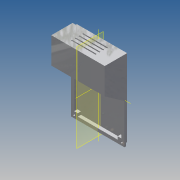
# Autodesk Inventor part: deksel
Saved by Autodesk Inventor 2020.4 (Build 244396000, 396)
## iProperties
Created: 2022-05-18
Part Number: deksel
Material: PC/ABS Plastic
Document SubType Name: Modeling
Designer: Lukas
Density: 0.357273 g/cm^3
Appearance: Smooth - White
Author: Lukas
Autodesk Inventor part; units mm, degrees
ref_plane "XZ Plane" through (0, 0, 0) normal (0, 1, 0) x (-1, 0, 0)
ref_plane "XY Plane" through (0, 0, 0) normal (0, 0, 1) x (1, 0, 0)
sketch "Sketch1" plane through (0, 0, 0) normal (0, 0, 1) x (1, 0, 0)
  line L0 (0, 105) -> (0, -105) projected
  line L1 (-70, 0) -> (70, 0) projected
  line L2 (-50, 75) -> (50, 75)
  line L3 (50, 75) -> (50, -75)
  line L4 (50, -75) -> (-50, -75)
  line L5 (-50, -75) -> (-50, 75)
  line L6 (-44, 69) -> (44, 69)
  line L7 (44, 69) -> (44, -69)
  line L8 (44, -69) -> (-44, -69)
  line L9 (-44, -69) -> (-44, 69)
  point P0 (0, 75)
  point P1 (50, 0)
  dimension "d1" = 100
  dimension "d2" = 150
  dimension "d3" = 6
  dimension "d4" = 6
  dimension "d5" = 6
  dimension "d6" = 6
  constraints: 16 end point, 4 parallel, 2 horizontal, 2 midpoint, 2 perpendicular, 2 point on line
  measures "d1" distance of L3.end L4.end
  measures "d2" distance of L2.end L3.end
  measures "d3" distance between parallel lines of L2 L6
  measures "d4" distance between parallel lines of L3 L7
  measures "d5" distance between parallel lines of L5 L9
  measures "d6" distance between parallel lines of L4 L8
extrude "Extrusion1" add sketch "Sketch1" along normal mid plane 3 contours L2 L3 L1 L7 L6 L0 | L0 L6 L9 L1 L5 L2 | L1 L9 L8 L0 L4 L5 | L3 L4 L0 L8 L7 L1
sketch "Sketch2" plane through (0, 0, -1.5) normal (0, 0, -1) x (-1, 0, 0)
  line L0 (-44, -69) -> (-44, 69) construction
  line L1 (-44, 69) -> (44, 69) construction
  line L2 (44, 69) -> (44, -69) construction
  line L3 (44, -69) -> (-44, -69) construction
  line L4 (44, -69) -> (44, 69) construction
  line L5 (-44, 69) -> (44, 69)
  line L6 (44, 69) -> (44, -69)
  line L7 (44, -69) -> (-44, -69)
  line L8 (-44, -69) -> (-44, 69)
  line L9 (47, -72) -> (-47, -72)
  line L10 (-47, -72) -> (-47, 72)
  line L11 (-47, 72) -> (47, 72)
  line L12 (47, 72) -> (47, -72)
  point P0 (0, 0)
  dimension "d9" = 3
  dimension "d10" = 3
  dimension "d11" = 3
  dimension "d12" = 3
  constraints: 16 end point, 4 parallel, 2 horizontal, 2 perpendicular
  measures "d9" distance between parallel lines of L11 L1
  measures "d10" distance between parallel lines of L10 L0
  measures "d11" distance between parallel lines of L12 L2
  measures "d12" distance between parallel lines of L3 L9
extrude "Extrusion2" add sketch "Sketch2" along normal blind 5
sketch "Sketch4" plane through (50, -75, 1.5) normal (1, 0, 0) x (0, 0, -1)
  line L0 (0, 0) -> (0, 150) construction
  line L1 (0, 0) -> (45, 0) construction
  line L2 (0, 150) -> (0, 0) construction
  line L3 (0, 75) -> (-36.8618, 100.8109)
  line L4 (0, 75) -> (45, 75) construction
  line L5 (0, 150) -> (-36.8618, 150)
  line L6 (-36.8618, 150) -> (-36.8618, 100.8109)
  line L7 (0, 75) -> (0, 150)
  line L8 (3, 0) -> (3, 150) construction
  line L9 (-3, 147) -> (-33.8618, 147)
  line L10 (-33.8618, 147) -> (-33.8618, 102.3726)
  line L11 (-33.8618, 102.3726) -> (-3, 80.7629)
  line L12 (-3, 147) -> (-3, 80.7629)
  line L13 (3, 0) -> (0, 0) construction
  line L14 (0, 78.6623) -> (3, 78.6623)
  line L15 (3, 78.6623) -> (3, 0)
  line L16 (3, 0) -> (0, 0)
  line L17 (0, 0) -> (0, 78.6623)
  point P0 (1.5, 75)
  dimension "d27" = 45
  dimension "d28" = 145
  dimension "d29" = 3
  dimension "d30" = 3
  dimension "d31" = 3
  dimension "d32" = 3
  constraints: 28 end point, 4 horizontal, 4 parallel, 4 perpendicular, 1 equal length, 1 midpoint, 1 point on line, 1 vertical
  measures "d27" distance of L3.start L3.end
  measures "d28" angle of L4 L3
  measures "d29" distance between parallel lines of L6 L10
  measures "d30" distance between parallel lines of L5 L9
  measures "d31" distance between parallel lines of L12 L0
  measures "d32" distance between parallel lines of L3 L11
extrude "Extrusion4" add sketch "Sketch4" against normal blind 100 contours L3 L6 L5 L7
sketch "Sketch5" plane through (47, -72, -1.5) normal (1, 0, 0) x (0, 0, -1)
  line L0 (0, 144) -> (0, 0) construction
  line L1 (5, 0) -> (5, 144) construction
  line L2 (0, 77.7875) -> (5, 77.7875)
  line L3 (5, 77.7875) -> (5, 0)
  line L4 (5, 0) -> (0, 0)
  line L5 (0, 0) -> (0, 77.7875)
  point P0 (-1.5, 72)
  constraints: 8 end point, 2 parallel, 1 horizontal, 1 perpendicular, 1 point on line
extrude "Extrusion5" add sketch "Sketch5" against normal blind 94
sketch "Sketch6" plane through (-44, 5.7875, -1.5) normal (0, 0, 1) x (1, 0, 0)
  line L0 (88, -74.7875) -> (0, -74.7875) construction
  line L1 (88, -5.7875) -> (0, -5.7875) construction
  line L2 (0, -74.7875) -> (88, -74.7875)
  line L3 (88, -74.7875) -> (88, -5.7875)
  line L4 (88, -5.7875) -> (0, -5.7875)
  line L5 (0, -5.7875) -> (0, -74.7875)
  point P0 (44, -5.7875)
  constraints: 8 end point, 2 parallel, 1 horizontal, 1 perpendicular
extrude "Extrusion6" cut sketch "Sketch6" against normal blind 3
sketch "Sketch7" plane through (50, -75, -1.5) normal (1, 0, 0) x (0, 0, -1)
  line L0 (-39.8618, 100.8109) -> (-3, 75) construction
  line L1 (-39.8618, 100.8109) -> (-39.8618, 150) construction
  line L2 (-3, 144) -> (-3, 75) construction
  line L3 (-39.8618, 150) -> (-3, 150)
  line L4 (-3, 150) -> (-3, 100.8109)
  line L5 (-39.8618, 100.8109) -> (-39.8618, 150)
  line L6 (-3, 75) -> (-39.8618, 100.8109) construction
  line L7 (-39.8618, 100.8109) -> (-3, 75)
  line L8 (-3, 75) -> (-3, 100.8109)
  point P0 (-1.5, 75)
  constraints: 10 end point, 2 equal length, 1 horizontal, 1 perpendicular, 1 point on line
extrude "Extrusion7" add sketch "Sketch7" against normal blind 1
sketch "Sketch8" plane through (44, 0, 1.5) normal (0, 0, -1) x (-1, 0, 0)
  line L0 (0, 5.7875) -> (0, 69) construction
  line L1 (88, 69) -> (0, 69)
  line L2 (0, 69) -> (0, 5.7875)
  line L3 (0, 5.7875) -> (88, 5.7875)
  line L4 (88, 5.7875) -> (88, 69)
  point P0 (44, 0)
  constraints: 8 end point, 2 parallel, 1 horizontal, 1 perpendicular
extrude "Extrusion8" cut sketch "Sketch8" against normal blind 3
sketch "Sketch9" plane through (-44, 5.7875, -1.5) normal (0, 0, 1) x (1, 0, 0)
  line L0 (88, -5.7875) -> (0, -5.7875) construction
  line L1 (88, -5.7875) -> (0, -5.7875)
  line L2 (0, -5.7875) -> (0, 0)
  line L3 (0, 0) -> (88, 0)
  line L4 (88, 0) -> (88, -5.7875)
  point P0 (44, -5.7875)
  constraints: 8 end point, 2 parallel, 1 horizontal, 1 perpendicular
extrude "Extrusion9" add sketch "Sketch9" along normal blind 3
sketch "Sketch10" plane through (-50, -75, -1.5) normal (-1, 0, 0) x (0, 0, 1)
  line L0 (3, 75) -> (39.8618, 100.8109) construction
  line L1 (0, 150) -> (39.8618, 150) construction
  line L2 (39.8618, 100.8109) -> (3, 100.8109)
  line L3 (3, 100.8109) -> (3, 150)
  line L4 (3, 150) -> (39.8618, 150)
  line L5 (39.8618, 150) -> (39.8618, 100.8109)
  line L6 (39.8618, 100.8109) -> (3, 75)
  line L7 (3, 75) -> (3, 6) construction
  line L8 (3, 100.8109) -> (3, 75)
  point P0 (1.5, 75)
  constraints: 12 end point, 3 equal length, 1 horizontal, 1 perpendicular, 1 point on line, 1 vertical
extrude "Extrusion10" add sketch "Sketch10" against normal blind 1
sketch "Sketch11" plane through (-50, 25.8109, 38.3618) normal (0, -0.8192, 0.5736) x (1, 0, 0)
  line L0 (100, 0) -> (0, 0) construction
  line L1 (100, -4.4392) -> (100, -90.4757) construction
  line L2 (0, 0) -> (100, 0)
  line L3 (100, 0) -> (100, -45)
  line L4 (100, -45) -> (0, -45)
  line L5 (3, -6.16) -> (3, -88.755) construction
  line L6 (0, -45) -> (0, 0)
  line L7 (0, -90.4757) -> (0, -4.4392) construction
  line L8 (25, -12.5) -> (65.2, -12.5)
  line L9 (65.2, -12.5) -> (65.2, -25.3)
  line L10 (65.2, -25.3) -> (25, -25.3)
  line L11 (25, -25.3) -> (25, -12.5)
  circle A0 centre (76.63, -18.9) radius 4
  point P0 (50, -46.2287)
  dimension "d48" = 40.2
  dimension "d49" = 12.8
  dimension "d51" = 25
  dimension "d52" = 8
  dimension "d53" = 11.43
  dimension "d71" = 12.5
  dimension "d72" = 18.9
  constraints: 16 end point, 3 perpendicular, 2 horizontal, 2 parallel, 1 centre point, 1 point on line
  measures "d48" distance of L9.end L10.end
  measures "d49" distance of L8.end L9.end
  measures "d51" distance between parallel lines of L7 L11
  measures "d52" diameter of A0
  measures "d53" distance from line of L9 A0.centre
  measures "d71" distance between parallel lines of L0 L8
  measures "d72" distance from line of L0 A0.centre
extrude "Extrusion11" cut sketch "Sketch11" against normal blind 3 contours L8 L9 L10 L11 | A0
sketch "Sketch12" plane through (-50, 75, -1.5) normal (0, 1, 0) x (1, 0, 0)
  line L0 (0, 0) -> (0, -39.8618) construction
  line L1 (100, -39.8618) -> (0, -39.8618) construction
  line L2 (100, -39.8618) -> (100, 0) construction
  line L3 (73.025, -29.8618) -> (26.975, -29.8618)
  line L4 (26.975, -29.8618) -> (26.975, -27.8618)
  line L5 (26.975, -27.8618) -> (73.025, -27.8618)
  line L6 (73.025, -27.8618) -> (73.025, -29.8618)
  line L7 (50, 13.9724) -> (50, -48.8342) construction
  line L8 (26.975, -22.8618) -> (73.025, -22.8618)
  line L9 (73.025, -22.8618) -> (73.025, -20.8618)
  line L10 (73.025, -20.8618) -> (26.975, -20.8618)
  line L11 (26.975, -20.8618) -> (26.975, -22.8618)
  line L12 (73.025, -15.8618) -> (26.975, -15.8618)
  line L13 (26.975, -15.8618) -> (26.975, -13.8618)
  line L14 (26.975, -13.8618) -> (73.025, -13.8618)
  line L15 (73.025, -13.8618) -> (73.025, -15.8618)
  line L16 (73.025, -8.8618) -> (26.975, -8.8618)
  line L17 (26.975, -8.8618) -> (26.975, -6.8618)
  line L18 (26.975, -6.8618) -> (73.025, -6.8618)
  line L19 (73.025, -6.8618) -> (73.025, -8.8618)
  point P0 (50, -1.5)
  point P1 (50, -29.8618)
  point P2 (50, -15.8618)
  point P3 (50, -8.8618)
  dimension "d56" = 26.975
  dimension "d57" = 2
  dimension "d58" = 10
  dimension "d59" = 5
  dimension "d60" = 2
  dimension "d61" = 26.975
  dimension "d62" = 26.975
  dimension "d63" = 5
  dimension "d64" = 2
  dimension "d65" = 26.975
  dimension "d66" = 5
  dimension "d67" = 26.975
  dimension "d68" = 2
  constraints: 32 end point, 8 parallel, 4 horizontal, 4 perpendicular, 3 midpoint, 3 point on line
  measures "d56" distance between parallel lines of L2 L6
  measures "d57" distance between parallel lines of L5 L3
  measures "d58" distance between parallel lines of L1 L3
  measures "d59" distance between parallel lines of L5 L8
  measures "d60" distance between parallel lines of L8 L10
  measures "d61" distance between parallel lines of L0 L11
  measures "d62" distance between parallel lines of L2 L9
  measures "d63" distance between parallel lines of L10 L12
  measures "d64" distance between parallel lines of L12 L14
  measures "d65" distance between parallel lines of L2 L15
  measures "d66" distance between parallel lines of L14 L16
  measures "d67" distance between parallel lines of L0 L17
  measures "d68" distance between parallel lines of L16 L18
extrude "Extrusion12" cut sketch "Sketch12" against normal blind 5
sketch "Sketch13" plane through (0, 0, -6.5) normal (0, 0, -1) x (-1, 0, 0)
  line L0 (-50, -75) -> (50, -75) construction
  line L1 (-50, 75) -> (-50, -75) construction
  line L2 (50, -75) -> (50, 75) construction
  point P0 (0, 0)
  point P1 (-44.5, -69.5)
  point P2 (44.5, -69.5)
  dimension "d73" = 5.5
  dimension "d74" = 5.5
  dimension "d75" = 5.5
  dimension "d76" = 5.5
  measures "d73" distance from line of L0 point (-44.5, -69.5)
  measures "d74" distance from line of L1 point (-44.5, -69.5)
  measures "d75" distance from line of L2 point (44.5, -69.5)
  measures "d76" distance from line of L0 point (44.5, -69.5)
hole "Hole1" at (44.5, -69.5, -6.5) at (-44.5, -69.5, -6.5) direction (0, 0, 1) diameter 4 end through all clearance for "Countersunk Flat Head Screw ISO 2009/7046" size "M4" standard "ISO"
sketch "Sketch14" plane through (0, 0, 1.5) normal (0, 0, 1) x (1, 0, 0)
  line L0 (-50, 0) -> (-50, -75) construction
  line L1 (-50, -75) -> (50, -75) construction
  line L2 (-44, -67.5635) -> (-44, 0) construction
  line L3 (-50, -63.5) -> (-38.5, -63.5)
  line L4 (-38.5, -63.5) -> (-38.5, -75)
  line L5 (-50, -63.5) -> (-50, -75)
  line L6 (-38.5, -75) -> (-50, -75)
  point P0 (0, 0)
  dimension "d84" = 11.5
  dimension "d85" = 11.5
  constraints: 8 end point, 2 collinear, 2 point on line, 1 horizontal, 1 perpendicular
  measures "d84" distance between parallel lines of L1 L3
  measures "d85" distance between parallel lines of L0 L4
extrude "Extrusion13" cut sketch "Sketch14" against normal blind 6
mirror "Mirror1" about plane through (0, 0, 0) normal (1, 0, 0) of "Extrusion13"
sketch "Sketch15" plane through (-44, 5.7875, -4.5) normal (0, 0, 1) x (1, 0, 0)
  line L0 (-6, -80.7875) -> (6.7524, -80.7875)
  line L1 (6.7524, -80.7875) -> (6.7524, -69.2875)
  line L2 (6.7524, -69.2875) -> (-6, -69.2875)
  line L3 (-6, -69.2875) -> (-6, -80.7875)
  line L4 (-6, -5.7875) -> (-6, -69.2875) construction
  line L5 (-6, -69.2875) -> (-6, 69.2125) construction
  line L6 (5.5, -80.7875) -> (82.5, -80.7875) construction
  point P0 (44, -5.7875)
  dimension "d88" = 0
  dimension "d89" = 0
  constraints: 8 end point, 2 parallel, 1 collinear, 1 horizontal, 1 perpendicular
  measures "d88" distance between parallel lines of L5 L3
  measures "d89" distance between parallel lines of L6 L0
extrude "Extrusion14" add sketch "Sketch15" along normal blind 6
mirror "Mirror2" about plane through (0, 0, 0) normal (1, 0, 0) of "Extrusion14"
sketch "Sketch16" plane through (-44.5, -69.5, -4.5) normal (0, 0, -1) x (-1, 0, 0)
  circle A0 centre (0, 0) radius 2 construction
  circle A1 centre (-89, 0) radius 2 construction
  point P0 (-44.5, 69.5)
  constraints: 2 coincident
hole "Hole2" at (-44.5, -69.5, -4.5) at (44.5, -69.5, -4.5) direction (0, 0, 1) diameter 4 end through all clearance for "Countersunk Flat Head Screw ISO 2009/7046" size "M4" standard "ISO"
sketch "Sketch17" plane through (50, -75, -4.5) normal (0, 0, -1) x (-1, 0, 0)
  line L0 (3, 11.5) -> (3, 3) construction
  line L1 (3, 11.5) -> (0, 11.5) construction
  line L2 (12.7524, 0) -> (12.7524, 3) construction
  line L3 (12.7524, 3) -> (12.7524, 0)
  line L4 (0, 0) -> (100, 0) construction
  line L5 (0, 0) -> (12.7524, 0)
  line L6 (0, 0) -> (0, 11.5)
  line L7 (0, 0) -> (0, 75) construction
  line L8 (0, 11.5) -> (3, 11.5) construction
  line L9 (3, 11.5) -> (0, 11.5)
  line L10 (0, 11.5) -> (3, 11.5)
  line L11 (3, 147) -> (3, 3) construction
  line L12 (3, 3) -> (12.7524, 3)
  line L13 (3, 3) -> (97, 3) construction
  line L14 (3, 3) -> (3, 11.5)
  point P0 (50, 75)
  constraints: 14 end point, 7 collinear
extrude "Extrusion15" cut sketch "Sketch17" against normal blind 3
mirror "Mirror3" about plane through (0, 0, 0) normal (1, 0, 0) of "Extrusion15"
body "Solid1"
